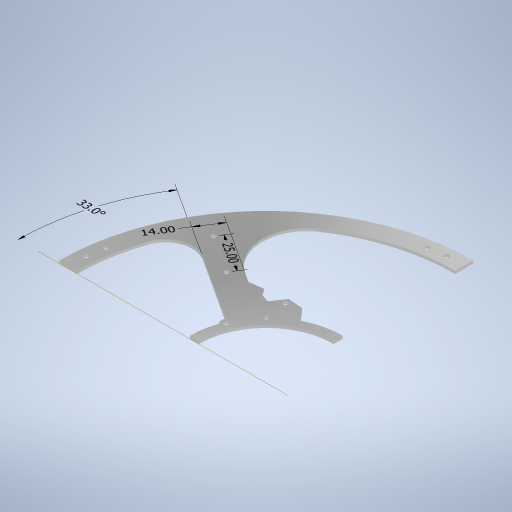
# Autodesk Inventor part: body_plate
Saved by Autodesk Inventor 2024.1 (Build 281209000, 209)
## iProperties
Created: 2024-08-02
Part Number: body_plate
Material: アルミニウム 6061
Document SubType Name: Sheet Metal
Designer: hibik
Density: 2.7 g/cm^3
Appearance: アルミニウム - フラット
Sheet Metal Rule: Default_mm
Author: hibik
Autodesk Inventor part; units mm, degrees
ref_plane "YZ Plane" through (0, 0, 0) normal (1, 0, 0) x (0, 1, 0)
ref_plane "XZ Plane" through (0, 0, 0) normal (0, 1, 0) x (-1, 0, 0)
ref_plane "XY Plane" through (0, 0, 0) normal (0, 0, 1) x (1, 0, 0)
sketch "スケッチ1" plane through (0, 0, 0) normal (0, 1, 0) x (-1, 0, 0)
  circle A0 centre (0, 0) radius 67
  circle A1 centre (0, 0) radius 62
  circle A2 centre (0, 0) radius 115
  circle A3 centre (0, 0) radius 105
  dimension "d0" = 134
  dimension "d1" = 124
  dimension "d2" = 230
  dimension "d5" = 210
  constraints: 4 centre point, 4 coincident
  measures "d0" diameter of A0
  measures "d1" diameter of A1
  measures "d2" diameter of A2
  measures "d5" diameter of A3
extrude "押し出し1" add sketch "スケッチ1" along normal blind 1.5
sketch "スケッチ2" plane through (0, 0, 0) normal (0, -1, 0) x (1, 0, 0)
  line L0 (40.8211, -35.6706) -> (45.1461, -32.6728) projected
  line L1 (45.1461, -32.6728) -> (44.7842, -28.2962) projected
  arc A0 (44.7842, -28.2962) -> (43.4491, -27.9248) centre (43.6139, -29.918) ccw projected
  line L2 (43.4491, -27.9248) -> (41.9542, -28.0485) projected
  arc A1 (41.9542, -28.0485) -> (38.889, -32.5383) centre (42.2426, -31.5365) ccw projected
  line L3 (38.889, -32.5383) -> (39.4183, -34.3101) projected
  arc A2 (39.4183, -34.3101) -> (40.8211, -35.6706) centre (41.3346, -33.7377) ccw projected
  circle A3 centre (42.2426, -31.5365) radius 1.35 projected
  arc A4 (20.2759, -44.9821) -> (16.4994, -41.7824) centre (16.7878, -45.2705) ccw projected
  line L4 (20.2759, -44.9821) -> (19.699, -38.0059) projected
  arc A5 (19.699, -38.0059) -> (15.9225, -34.8062) centre (16.2109, -38.2943) ccw projected
  line L5 (15.9225, -34.8062) -> (12.4344, -35.0947) projected
  line L6 (12.4344, -35.0947) -> (13.0113, -42.0709) projected
  line L7 (13.0113, -42.0709) -> (16.4994, -41.7824) projected
  circle A6 centre (16.2109, -38.2943) radius 1.35 projected
  line L8 (-32.6728, -45.1461) -> (-28.2962, -44.7842) projected
  arc A7 (-28.2962, -44.7842) -> (-27.9248, -43.4491) centre (-29.918, -43.6139) ccw projected
  line L9 (-27.9248, -43.4491) -> (-28.0485, -41.9542) projected
  arc A8 (-28.0485, -41.9542) -> (-32.5383, -38.889) centre (-31.5365, -42.2426) ccw projected
  line L10 (-32.5383, -38.889) -> (-34.3101, -39.4183) projected
  arc A9 (-34.3101, -39.4183) -> (-35.6706, -40.8211) centre (-33.7377, -41.3346) ccw projected
  line L11 (-35.6706, -40.8211) -> (-32.6728, -45.1461) projected
  circle A10 centre (-31.5365, -42.2426) radius 1.35 projected
  arc A11 (-44.9821, -20.2759) -> (-41.7824, -16.4994) centre (-45.2705, -16.7878) ccw projected
  line L12 (-44.9821, -20.2759) -> (-38.0059, -19.699) projected
  arc A12 (-38.0059, -19.699) -> (-34.8062, -15.9225) centre (-38.2943, -16.2109) ccw projected
  line L13 (-34.8062, -15.9225) -> (-35.0947, -12.4344) projected
  line L14 (-35.0947, -12.4344) -> (-42.0709, -13.0113) projected
  line L15 (-42.0709, -13.0113) -> (-41.7824, -16.4994) projected
  circle A13 centre (-38.2943, -16.2109) radius 1.35 projected
  arc A14 (-20.2759, 44.9821) -> (-16.4994, 41.7824) centre (-16.7878, 45.2705) ccw projected
  line L16 (-20.2759, 44.9821) -> (-19.699, 38.0059) projected
  arc A15 (-19.699, 38.0059) -> (-15.9225, 34.8062) centre (-16.2109, 38.2943) ccw projected
  line L17 (-15.9225, 34.8062) -> (-12.4344, 35.0947) projected
  line L18 (-12.4344, 35.0947) -> (-13.0113, 42.0709) projected
  line L19 (-13.0113, 42.0709) -> (-16.4994, 41.7824) projected
  circle A16 centre (-16.2109, 38.2943) radius 1.35 projected
  line L20 (35.6706, 40.8211) -> (32.6728, 45.1461) projected
  line L21 (32.6728, 45.1461) -> (28.2962, 44.7842) projected
  arc A17 (28.2962, 44.7842) -> (27.9248, 43.4491) centre (29.918, 43.6139) ccw projected
  line L22 (27.9248, 43.4491) -> (28.0485, 41.9542) projected
  arc A18 (28.0485, 41.9542) -> (32.5383, 38.889) centre (31.5365, 42.2426) ccw projected
  line L23 (32.5383, 38.889) -> (34.3101, 39.4183) projected
  arc A19 (34.3101, 39.4183) -> (35.6706, 40.8211) centre (33.7377, 41.3346) ccw projected
  circle A20 centre (31.5365, 42.2426) radius 1.35 projected
  circle A21 centre (-42.2426, 31.5365) radius 1.35 projected
  line L24 (-40.8211, 35.6706) -> (-45.1461, 32.6728) projected
  line L25 (-45.1461, 32.6728) -> (-44.7842, 28.2962) projected
  arc A22 (-44.7842, 28.2962) -> (-43.4491, 27.9248) centre (-43.6139, 29.918) ccw projected
  line L26 (-43.4491, 27.9248) -> (-41.9542, 28.0485) projected
  arc A23 (-41.9542, 28.0485) -> (-38.889, 32.5383) centre (-42.2426, 31.5365) ccw projected
  line L27 (-38.889, 32.5383) -> (-39.4183, 34.3101) projected
  arc A24 (-39.4183, 34.3101) -> (-40.8211, 35.6706) centre (-41.3346, 33.7377) ccw projected
  arc A25 (44.9821, 20.2759) -> (41.7824, 16.4994) centre (45.2705, 16.7878) ccw projected
  line L28 (44.9821, 20.2759) -> (38.0059, 19.699) projected
  arc A26 (38.0059, 19.699) -> (34.8062, 15.9225) centre (38.2943, 16.2109) ccw projected
  line L29 (34.8062, 15.9225) -> (35.0947, 12.4344) projected
  line L30 (35.0947, 12.4344) -> (42.0709, 13.0113) projected
  line L31 (42.0709, 13.0113) -> (41.7824, 16.4994) projected
  circle A27 centre (38.2943, 16.2109) radius 1.35 projected
  circle A28 centre (0, 0) radius 37.5
  line L32 (16.9004, -64.8335) -> (16.4816, -59.7692) projected
  arc A29 (16.9004, -64.8335) -> (45.2274, -49.4315) centre (0, 0) ccw projected
  line L33 (44.838, -44.7223) -> (45.2274, -49.4315) projected
  arc A30 (39.1412, -40.3701) -> (44.838, -44.7223) centre (44.986, -38.6241) ccw projected
  line L34 (36.9727, -33.1108) -> (39.1412, -40.3701) projected
  arc A31 (41.7893, -26.0553) -> (36.9727, -33.1108) centre (42.2426, -31.5365) ccw projected
  line L35 (45.2774, -25.7668) -> (41.7893, -26.0553) projected
  line L36 (45.2319, -25.2161) -> (45.2774, -25.7668) projected
  line L37 (45.2319, -25.2161) -> (29.6057, -11.9768) projected
  arc A32 (16.6771, -27.2363) -> (29.6057, -11.9768) centre (0, 0) ccw projected
  line L38 (16.6771, -27.2363) -> (40.2207, -47.1836) projected
  arc A33 (16.4816, -59.7692) -> (40.2207, -47.1836) centre (0, 0) ccw projected
  line L39 (-64.8335, -16.9004) -> (-59.7692, -16.4816) projected
  arc A34 (-64.8335, -16.9004) -> (-49.4315, -45.2274) centre (0, 0) ccw projected
  line L40 (-44.7223, -44.838) -> (-49.4315, -45.2274) projected
  arc A35 (-40.3701, -39.1412) -> (-44.7223, -44.838) centre (-38.6241, -44.986) ccw projected
  line L41 (-33.1108, -36.9727) -> (-40.3701, -39.1412) projected
  arc A36 (-26.0553, -41.7893) -> (-33.1108, -36.9727) centre (-31.5365, -42.2426) ccw projected
  line L42 (-25.9316, -43.2842) -> (-26.0553, -41.7893) projected
  line L43 (-23.3877, -43.0739) -> (-25.9316, -43.2842) projected
  line L44 (-23.3877, -43.0739) -> (-11.9768, -29.6057) projected
  arc A37 (-27.2363, -16.6771) -> (-11.9768, -29.6057) centre (0, 0) ccw projected
  line L45 (-27.2363, -16.6771) -> (-47.1836, -40.2207) projected
  arc A38 (-59.7692, -16.4816) -> (-47.1836, -40.2207) centre (0, 0) ccw projected
  line L46 (-16.9004, 64.8335) -> (-16.4816, 59.7692) projected
  arc A39 (-16.9004, 64.8335) -> (-45.2274, 49.4315) centre (0, 0) ccw projected
  line L47 (-44.838, 44.7223) -> (-45.2274, 49.4315) projected
  arc A40 (-39.1412, 40.3701) -> (-44.838, 44.7223) centre (-44.986, 38.6241) ccw projected
  line L48 (-36.9727, 33.1108) -> (-39.1412, 40.3701) projected
  arc A41 (-41.7893, 26.0553) -> (-36.9727, 33.1108) centre (-42.2426, 31.5365) ccw projected
  line L49 (-43.2842, 25.9316) -> (-41.7893, 26.0553) projected
  line L50 (-43.0739, 23.3877) -> (-43.2842, 25.9316) projected
  line L51 (-43.0739, 23.3877) -> (-29.6057, 11.9768) projected
  arc A42 (-16.6771, 27.2363) -> (-29.6057, 11.9768) centre (0, 0) ccw projected
  line L52 (-16.6771, 27.2363) -> (-40.2207, 47.1836) projected
  arc A43 (-16.4816, 59.7692) -> (-40.2207, 47.1836) centre (0, 0) ccw projected
  line L53 (64.8335, 16.9004) -> (59.7692, 16.4816) projected
  arc A44 (64.8335, 16.9004) -> (49.4315, 45.2274) centre (0, 0) ccw projected
  line L54 (44.7223, 44.838) -> (49.4315, 45.2274) projected
  arc A45 (40.3701, 39.1412) -> (44.7223, 44.838) centre (38.6241, 44.986) ccw projected
  line L55 (33.1108, 36.9727) -> (40.3701, 39.1412) projected
  arc A46 (26.0553, 41.7893) -> (33.1108, 36.9727) centre (31.5365, 42.2426) ccw projected
  line L56 (25.9316, 43.2842) -> (26.0553, 41.7893) projected
  line L57 (23.3877, 43.0739) -> (25.9316, 43.2842) projected
  line L58 (23.3877, 43.0739) -> (11.9768, 29.6057) projected
  arc A47 (27.2363, 16.6771) -> (11.9768, 29.6057) centre (0, 0) ccw projected
  line L59 (27.2363, 16.6771) -> (47.1836, 40.2207) projected
  arc A48 (59.7692, 16.4816) -> (47.1836, 40.2207) centre (0, 0) ccw projected
  circle A49 centre (0, 0) radius 42.5
  line L60 (10.8533, -40.2425) -> (13.0113, -42.0709) projected
  line L61 (6.3617, -40.6139) -> (6.5265, -42.6071) projected
  line L62 (-40.6139, -6.3617) -> (-42.6071, -6.5265) projected
  line L63 (-6.3617, 40.6139) -> (-6.5265, 42.6071) projected
  line L64 (31.4411, 5.6032) -> (42.6071, 6.5265) projected
  line L65 (40.8211, -35.6706) -> (38.2663, -37.4414)
  line L66 (44.7842, -28.2962) -> (44.4766, -24.5762)
  line L67 (35.6706, 40.8211) -> (37.4414, 38.2663)
  line L68 (28.2962, 44.7842) -> (24.5762, 44.4766)
  line L69 (-40.8211, 35.6706) -> (-38.2663, 37.4414)
  line L70 (-44.7842, 28.2962) -> (-44.4766, 24.5762)
  line L71 (-35.6706, -40.8211) -> (-37.4414, -38.2663)
  line L72 (-28.2962, -44.7842) -> (-24.5762, -44.4766)
  line L73 (-25.2161, -45.2319) -> (-23.3877, -43.0739) projected
  line L74 (-45.2319, 25.2161) -> (-43.0739, 23.3877) projected
  line L75 (25.2161, 45.2319) -> (23.3877, 43.0739) projected
  circle A50 centre (-16.2109, 38.2943) radius 3
  circle A51 centre (-38.2943, -16.2109) radius 3
  circle A52 centre (16.2109, -38.2943) radius 3
  circle A53 centre (38.2943, 16.2109) radius 3
  point P0 (40.1725, 13.8716)
  point P1 (37.922, 19.1878)
  point P2 (-13.8716, 40.1725)
  point P3 (-19.1878, 37.922)
  point P4 (-25.0517, 34.3317)
  point P5 (-37.9803, 19.0722)
  point P6 (-40.1725, -13.8716)
  point P7 (-37.922, -19.1878)
  point P8 (-34.3317, -25.0517)
  point P9 (-19.0722, -37.9803)
  point P10 (13.8716, -40.1725)
  point P11 (19.1878, -37.922)
  point P12 (25.0517, -34.3317)
  point P13 (37.9803, -19.0722)
  point P14 (19.0722, 37.9803)
  point P15 (34.3317, 25.0517)
  dimension "d6" = 75
  dimension "d7" = 85
  dimension "d10" = 360
  dimension "d12" = 6
  dimension "d13" = 6
  dimension "d14" = 6
  dimension "d15" = 6
  constraints: 16 end point, 6 centre point, 6 coincident, 2 collinear, 2 point on line, 25 other
  measures "d6" diameter of A28
  measures "d7" diameter of A49
  measures "d12" diameter of A50
  measures "d13" diameter of A51
  measures "d14" diameter of A52
  measures "d15" diameter of A53
extrude "押し出し2" add sketch "スケッチ2" against normal up to surface (1.5 mm away) contours A2 L3 A1 L2 A0 L1 L0 | L65 L34 A31 L35 L66 A0 L2 A1 L3 A2 | L34 A30 L33 A29 L32 A33 L38 A49 L37 L66 L35 A31 | A49 L38 A28 L37 | L37 A28 L64 A49 | A49 A5 L5 A28 L38 | A49 A52 L6 A28 L5 A5 | L64 A28 L30 A49 | A52 A49 A6 | A49 A6 A52 | L30 A28 L29 A26 A49 A53 | L6 A49 L44 A28 | A53 A49 A27 | A49 A27 A53 | L44 A49 L45 A28 | A28 L59 A49 A26 L29 | L45 A49 A12 L13 A28 | L44 L43 L42 A36 L41 A35 L40 A34 L39 A38 L45 A49 | A28 L58 A49 L59 | L13 A12 A49 A51 L14 A28 | L73 L72 A7 L9 A8 L10 A9 L71 L41 A36 L42 L43 | A28 L18 A49 L58 | A49 L58 L57 L56 A46 L55 A45 L54 A44 L53 A48 L59 | L14 A49 L51 A28 | A28 L17 A15 A49 A50 L18 | L51 A49 L52 A28 | A51 A49 A13 | A49 A13 A51 | L8 L11 A9 L10 A8 L9 A7 | A28 L52 A49 A15 L17 | L75 L68 A17 L22 A18 L23 A19 L67 L55 A46 L56 L57 | L51 L50 L49 A41 L48 A40 L47 A39 L46 A43 L52 A49 | A50 A49 A16 | A49 A16 A50 | L74 L70 A22 L26 A23 L27 A24 L69 L48 A41 L49 L50 | L21 L20 A19 L23 A18 L22 A17 | L25 L24 A24 L27 A23 L26 A22
sketch "スケッチ3" plane through (0, 0, 0) normal (0, -1, 0) x (1, 0, 0)
  line L0 (-63.0578, 84.2479) -> (51.3164, -91.8729)
  line L1 (51.3164, -91.8729) -> (63.0578, -84.2479) construction
  line L2 (63.0578, -84.2479) -> (-51.3164, 91.8729)
  line L3 (-51.3164, 91.8729) -> (-63.0578, 84.2479) construction
  line L4 (-63.0578, 84.2479) -> (63.0578, -84.2479) construction
  line L5 (51.3164, -91.8729) -> (-51.3164, 91.8729) construction
  line L6 (91.8729, 51.3164) -> (-84.2479, -63.0578)
  line L7 (-84.2479, -63.0578) -> (-91.8729, -51.3164) construction
  line L8 (-91.8729, -51.3164) -> (84.2479, 63.0578)
  line L9 (84.2479, 63.0578) -> (91.8729, 51.3164) construction
  circle A0 centre (0, 0) radius 105 projected
  line L10 (91.8729, 51.3164) -> (-91.8729, -51.3164) construction
  line L11 (-84.2479, -63.0578) -> (84.2479, 63.0578) construction
  line L12 (0, -161) -> (0, 161) projected
  circle A1 centre (0, 0) radius 67 projected
  arc A2 (-44.4604, -43.2119) -> (40.2207, -47.1836) centre (0, 0) ccw projected
  arc A3 (-40.3701, -39.1412) -> (-44.4604, -43.2119) centre (-38.6241, -44.986) ccw projected
  line L13 (-40.3701, -39.1412) -> (-37.4414, -38.2663) projected
  line L14 (-37.4414, -38.2663) -> (-32.6728, -45.1461) projected
  line L15 (-32.6728, -45.1461) -> (-24.5762, -44.4766) projected
  line L16 (-24.5762, -44.4766) -> (-19.0722, -37.9803) projected
  arc A4 (-19.0722, -37.9803) -> (13.8716, -40.1725) centre (0, 0) ccw projected
  arc A5 (13.8716, -40.1725) -> (19.1878, -37.922) centre (16.2109, -38.2943) ccw projected
  arc A6 (19.1878, -37.922) -> (25.0517, -34.3317) centre (0, 0) ccw projected
  line L17 (25.0517, -34.3317) -> (40.2207, -47.1836) projected
  arc A7 (39.1412, -40.3701) -> (43.2119, -44.4604) centre (44.986, -38.6241) ccw projected
  line L18 (39.1412, -40.3701) -> (38.2663, -37.4414) projected
  line L19 (38.2663, -37.4414) -> (45.1461, -32.6728) projected
  line L20 (45.1461, -32.6728) -> (44.4766, -24.5762) projected
  line L21 (44.4766, -24.5762) -> (37.9803, -19.0722) projected
  arc A8 (37.9803, -19.0722) -> (40.1725, 13.8716) centre (0, 0) ccw projected
  arc A9 (40.1725, 13.8716) -> (37.922, 19.1878) centre (38.2943, 16.2109) ccw projected
  arc A10 (37.922, 19.1878) -> (34.3317, 25.0517) centre (0, 0) ccw projected
  arc A11 (-13.8716, 40.1725) -> (-19.1878, 37.922) centre (-16.2109, 38.2943) ccw projected
  arc A12 (-19.1878, 37.922) -> (-25.0517, 34.3317) centre (0, 0) ccw projected
  line L22 (-25.0517, 34.3317) -> (-40.2207, 47.1836) projected
  arc A13 (44.4604, 43.2119) -> (-40.2207, 47.1836) centre (0, 0) ccw projected
  circle A14 centre (0, 0) radius 37.5 projected
  circle A15 centre (42.2426, -31.5365) radius 1.35 projected
  circle A16 centre (16.2109, -38.2943) radius 1.35 projected
  circle A17 centre (-38.2943, -16.2109) radius 1.35 projected
  circle A18 centre (-16.2109, 38.2943) radius 1.35 projected
  circle A19 centre (38.2943, 16.2109) radius 1.35 projected
  circle A20 centre (-42.2426, 31.5365) radius 1.35 projected
  circle A21 centre (-31.5365, -42.2426) radius 1.35 projected
  arc A22 (-39.1412, 40.3701) -> (-43.2119, 44.4604) centre (-44.986, 38.6241) ccw projected
  line L23 (-39.1412, 40.3701) -> (-38.2663, 37.4414) projected
  line L24 (-38.2663, 37.4414) -> (-45.1461, 32.6728) projected
  line L25 (-45.1461, 32.6728) -> (-44.4766, 24.5762) projected
  line L26 (-44.4766, 24.5762) -> (-37.9803, 19.0722) projected
  arc A23 (-37.9803, 19.0722) -> (-40.1725, -13.8716) centre (0, 0) ccw projected
  arc A24 (-40.1725, -13.8716) -> (-37.922, -19.1878) centre (-38.2943, -16.2109) ccw projected
  arc A25 (-37.922, -19.1878) -> (-34.3317, -25.0517) centre (0, 0) ccw projected
  line L27 (-34.3317, -25.0517) -> (-47.1836, -40.2207) projected
  arc A26 (-43.2119, 44.4604) -> (-47.1836, -40.2207) centre (0, 0) ccw projected
  circle A27 centre (0, 0) radius 67 projected
  line L28 (34.3317, 25.0517) -> (47.1836, 40.2207) projected
  arc A28 (43.2119, -44.4604) -> (47.1836, 40.2207) centre (0, 0) ccw projected
  arc A29 (40.3701, 39.1412) -> (44.4604, 43.2119) centre (38.6241, 44.986) ccw projected
  line L29 (40.3701, 39.1412) -> (37.4414, 38.2663) projected
  line L30 (37.4414, 38.2663) -> (32.6728, 45.1461) projected
  line L31 (32.6728, 45.1461) -> (24.5762, 44.4766) projected
  line L32 (24.5762, 44.4766) -> (19.0722, 37.9803) projected
  arc A30 (19.0722, 37.9803) -> (-13.8716, 40.1725) centre (0, 0) ccw projected
  point P0 (42.1618, -52.0709)
  point P1 (30.4204, -59.6959)
  point P2 (51.1892, -91.677)
  point P3 (62.9306, -84.052)
  point P4 (18.0575, -40.6587)
  point P5 (27.681, -55.4776)
  point P6 (-52.0709, -42.1618)
  point P7 (-59.6959, -30.4204)
  point P8 (-91.677, -51.1892)
  point P9 (-84.052, -62.9306)
  point P10 (-40.6587, -18.0575)
  point P11 (-55.4776, -27.681)
  point P12 (-42.1618, 52.0709)
  point P13 (-30.4204, 59.6959)
  point P14 (-51.1892, 91.677)
  point P15 (-62.9306, 84.052)
  point P16 (-18.0575, 40.6587)
  point P17 (-27.681, 55.4776)
  point P18 (40.6587, 18.0575)
  point P19 (55.4776, 27.681)
  point P20 (52.0709, 42.1618)
  point P21 (59.6959, 30.4204)
  point P22 (91.677, 51.1892)
  point P23 (84.052, 62.9306)
  dimension "d18" = 14
  dimension "d19" = 33
  constraints: 24 end point, 4 midpoint, 4 parallel, 4 perpendicular, 2 tangent
  measures "d18" distance between parallel lines of L2 L0
  measures "d19" angle of L0 L12
extrude "押し出し3" add sketch "スケッチ3" against normal up to surface (1.5 mm away) contours A0 L2 A1 L0 | L8 A1 L6 A0 | A13 L2 A11 A12 L22 L0 | L0 L22 A13 | L8 A24 A25 L27 L6 A26 | A0 L6 A1 L8 | L6 L27 A26 | L0 A1 L2 A0 | A28 L6 A9 A10 L28 L8 | L8 L28 A28 | L0 A5 A6 L17 L2 A2 | L2 L17 A2
sketch "スケッチ4" plane through (0, 0, 0) normal (0, -1, 0) x (1, 0, 0)
  arc A0 (52.0709, 42.1618) -> (-30.4204, 59.6959) centre (0, 0) ccw projected
  line L0 (-30.4204, 59.6959) -> (-51.1892, 91.677) projected
  arc A1 (84.052, 62.9306) -> (-51.1892, 91.677) centre (0, 0) ccw projected
  line L1 (84.052, 62.9306) -> (52.0709, 42.1618) projected
  line L2 (59.6959, 30.4204) -> (91.677, 51.1892) projected
  arc A2 (62.9306, -84.052) -> (91.677, 51.1892) centre (0, 0) ccw projected
  line L3 (62.9306, -84.052) -> (42.1618, -52.0709) projected
  arc A3 (42.1618, -52.0709) -> (59.6959, 30.4204) centre (0, 0) ccw projected
  arc A4 (-42.1618, 52.0709) -> (-59.6959, -30.4204) centre (0, 0) ccw projected
  line L4 (-59.6959, -30.4204) -> (-91.677, -51.1892) projected
  arc A5 (-62.9306, 84.052) -> (-91.677, -51.1892) centre (0, 0) ccw projected
  line L5 (-62.9306, 84.052) -> (-42.1618, 52.0709) projected
  circle A6 centre (0, 0) radius 115 projected
  arc A7 (-43.2119, 44.4604) -> (-55.4776, -27.681) centre (0, 0) ccw projected
  arc A8 (-39.1412, 40.3701) -> (-43.2119, 44.4604) centre (-44.986, 38.6241) ccw projected
  line L6 (-39.1412, 40.3701) -> (-38.2663, 37.4414) projected
  line L7 (-38.2663, 37.4414) -> (-45.1461, 32.6728) projected
  line L8 (-45.1461, 32.6728) -> (-44.4766, 24.5762) projected
  line L9 (-44.4766, 24.5762) -> (-37.9803, 19.0722) projected
  arc A9 (-37.9803, 19.0722) -> (-40.1725, -13.8716) centre (0, 0) ccw projected
  arc A10 (-40.1725, -13.8716) -> (-40.6587, -18.0575) centre (-38.2943, -16.2109) ccw projected
  line L10 (-40.6587, -18.0575) -> (-55.4776, -27.681) projected
  arc A11 (-40.3701, -39.1412) -> (-44.4604, -43.2119) centre (-38.6241, -44.986) ccw projected
  line L11 (-40.3701, -39.1412) -> (-37.4414, -38.2663) projected
  line L12 (-37.4414, -38.2663) -> (-32.6728, -45.1461) projected
  line L13 (-32.6728, -45.1461) -> (-24.5762, -44.4766) projected
  line L14 (-24.5762, -44.4766) -> (-19.0722, -37.9803) projected
  arc A12 (-19.0722, -37.9803) -> (13.8716, -40.1725) centre (0, 0) ccw projected
  arc A13 (13.8716, -40.1725) -> (18.0575, -40.6587) centre (16.2109, -38.2943) ccw projected
  line L15 (18.0575, -40.6587) -> (27.681, -55.4776) projected
  arc A14 (-44.4604, -43.2119) -> (27.681, -55.4776) centre (0, 0) ccw projected
  arc A15 (39.1412, -40.3701) -> (43.2119, -44.4604) centre (44.986, -38.6241) ccw projected
  line L16 (39.1412, -40.3701) -> (38.2663, -37.4414) projected
  line L17 (38.2663, -37.4414) -> (45.1461, -32.6728) projected
  line L18 (45.1461, -32.6728) -> (44.4766, -24.5762) projected
  line L19 (44.4766, -24.5762) -> (37.9803, -19.0722) projected
  arc A16 (37.9803, -19.0722) -> (40.1725, 13.8716) centre (0, 0) ccw projected
  arc A17 (40.1725, 13.8716) -> (40.6587, 18.0575) centre (38.2943, 16.2109) ccw projected
  line L20 (40.6587, 18.0575) -> (55.4776, 27.681) projected
  arc A18 (43.2119, -44.4604) -> (55.4776, 27.681) centre (0, 0) ccw projected
  circle A19 centre (0, 0) radius 37.5 projected
  circle A20 centre (42.2426, -31.5365) radius 1.35 projected
  circle A21 centre (16.2109, -38.2943) radius 1.35 projected
  circle A22 centre (-38.2943, -16.2109) radius 1.35 projected
  circle A23 centre (-16.2109, 38.2943) radius 1.35 projected
  circle A24 centre (38.2943, 16.2109) radius 1.35 projected
  circle A25 centre (-42.2426, 31.5365) radius 1.35 projected
  circle A26 centre (-31.5365, -42.2426) radius 1.35 projected
  circle A27 centre (31.5365, 42.2426) radius 1.35 projected
  arc A28 (40.3701, 39.1412) -> (44.4604, 43.2119) centre (38.6241, 44.986) ccw projected
  line L21 (40.3701, 39.1412) -> (37.4414, 38.2663) projected
  line L22 (37.4414, 38.2663) -> (32.6728, 45.1461) projected
  line L23 (32.6728, 45.1461) -> (24.5762, 44.4766) projected
  line L24 (24.5762, 44.4766) -> (19.0722, 37.9803) projected
  arc A29 (19.0722, 37.9803) -> (-13.8716, 40.1725) centre (0, 0) ccw projected
  arc A30 (-13.8716, 40.1725) -> (-18.0575, 40.6587) centre (-16.2109, 38.2943) ccw projected
  line L25 (-18.0575, 40.6587) -> (-27.681, 55.4776) projected
  arc A31 (44.4604, 43.2119) -> (-27.681, 55.4776) centre (0, 0) ccw projected
  line L26 (30.4204, -59.6959) -> (51.1892, -91.677) projected
  arc A32 (-84.052, -62.9306) -> (51.1892, -91.677) centre (0, 0) ccw projected
  line L27 (-84.052, -62.9306) -> (-52.0709, -42.1618) projected
  arc A33 (-52.0709, -42.1618) -> (30.4204, -59.6959) centre (0, 0) ccw projected
  line L28 (30.4204, -59.6959) -> (27.681, -55.4776)
  line L29 (-52.0709, -42.1618) -> (-44.4604, -43.2119)
  line L30 (42.1618, -52.0709) -> (43.2119, -44.4604)
  line L31 (59.6959, 30.4204) -> (55.4776, 27.681)
  line L32 (52.0709, 42.1618) -> (44.4604, 43.2119)
  line L33 (-30.4204, 59.6959) -> (-27.681, 55.4776)
  line L34 (-42.1618, 52.0709) -> (-43.2119, 44.4604)
  line L35 (-59.6959, -30.4204) -> (-55.4776, -27.681)
  circle A34 centre (62.9003, 40.8479) radius 1.3
  line L36 (62.9003, 40.8479) -> (0, 0) construction
  line L37 (62.9003, 40.8479) -> (64.3271, 38.6509) construction
  circle A35 centre (83.8671, 54.4639) radius 1.3
  line L38 (62.9003, 40.8479) -> (83.8671, 54.4639) construction
  circle A36 centre (-54.4639, 83.8671) radius 1.3
  circle A37 centre (-40.8479, 62.9003) radius 1.3
  circle A38 centre (-83.8671, -54.4639) radius 1.3
  circle A39 centre (-62.9003, -40.8479) radius 1.3
  circle A40 centre (54.4639, -83.8671) radius 1.3
  circle A41 centre (40.8479, -62.9003) radius 1.3
  point P0 (-30.4204, 59.6959)
  point P1 (44.4604, 43.2119)
  point P2 (-59.6959, -30.4204)
  dimension "d24" = 360
  dimension "d34" = 2.6
  dimension "d35" = 7
  dimension "d36" = 7
  dimension "d37" = 75
  dimension "d39" = 25
  dimension "d42" = 360
  constraints: 22 end point, 8 centre point, 2 coincident, 2 collinear, 1 equal radius, 1 perpendicular, 44 other
  measures "d34" diameter of A34
  measures "d35" distance from line of L1 L36.start
  measures "d36" distance from line of L2 L36.start
  measures "d37" distance from line of point (0, 0) L37
  measures "d39" distance from line of L38.end L37
extrude "押し出し4" cut sketch "スケッチ4" against normal through all contours L32 A31 L33 A0 | A3 L30 A18 L31 | L34 A7 L35 A4 | A14 L28 A33 L29 | A34 | A35 | A36 | A37 | A38 | A39 | A40 | A41
fillet "フィレット1" radius 25 4 edges at (62.9306, 0.75, -84.052) (84.052, 0.75, 62.9306) (-62.9306, 0.75, 84.052) (-84.052, 0.75, -62.9306)
fillet "フィレット2" radius 15 4 edges at (91.677, 0.75, 51.1892) (51.1892, 0.75, -91.677) (-91.677, 0.75, -51.1892) (-51.1892, 0.75, 91.677)
sketch "スケッチ5" plane through (0, 0, 0) normal (0, -1, 0) x (1, 0, 0)
  line L0 (30, 30) -> (-30, 30) construction
  line L1 (-30, 30) -> (-30, -30) construction
  line L2 (-30, -30) -> (30, -30) construction
  line L3 (30, -30) -> (30, 30) construction
  line L4 (30, 30) -> (-30, -30) construction
  line L5 (-30, 30) -> (30, -30) construction
  circle A0 centre (-30, 30) radius 1.3
  circle A1 centre (30, 30) radius 1.3
  circle A2 centre (30, -30) radius 1.3
  circle A3 centre (-30, -30) radius 1.3
  point P0 (0, 0)
  dimension "d30" = 2.6
  dimension "d31" = 60
  constraints: 12 end point, 4 centre point, 4 coincident, 3 equal radius, 2 midpoint, 2 parallel, 2 perpendicular, 1 horizontal
  measures "d30" diameter of A0
  measures "d31" distance of L0.start L0.end
extrude "押し出し5" cut sketch "スケッチ5" against normal through all
sketch "スケッチ6" plane through (0, 1.5, 0) normal (0, 1, 0) x (1, 0, 0)
  line L0 (0, 139.1279) -> (158.6637, 139.1279)
  line L1 (158.6637, 139.1279) -> (158.6637, -140)
  line L2 (158.6637, -140) -> (0, -140)
  line L3 (0, -140) -> (0, 139.1279)
  line L4 (-207.7572, 0) -> (158.6637, 0)
  line L5 (158.6637, 0) -> (158.6637, -140)
  line L6 (158.6637, -140) -> (-207.7572, -140)
  line L7 (-207.7572, -140) -> (-207.7572, 0)
  line L8 (0, 194.9535) -> (0, -195.8256) projected
  line L9 (-281.0413, 0) -> (231.9478, 0) projected
  point P0 (0, 0)
  point P1 (0, 0)
  constraints: 16 end point, 4 parallel, 3 collinear, 2 horizontal, 2 perpendicular, 1 point on line
extrude "押し出し6" cut sketch "スケッチ6" against normal through all
sketch "スケッチ7" plane through (0, 1.5, 0) normal (0, 1, 0) x (1, 0, 0)
  line L0 (0, 0) -> (-109.5814, 9.5871) construction
  line L1 (0, 0) -> (-108.3289, 19.1013) construction
  line L2 (0, 0) -> (-19.1013, 108.3289) construction
  line L3 (0, 0) -> (-9.5871, 109.5814) construction
  line L4 (0, 161) -> (0, -161) projected
  line L5 (-161, 0) -> (161, 0) projected
  circle A0 centre (0, 0) radius 110 construction
  circle A1 centre (-9.5871, 109.5814) radius 1.5
  circle A2 centre (-19.1013, 108.3289) radius 1.5
  circle A3 centre (-108.3289, 19.1013) radius 1.5
  circle A4 centre (-109.5814, 9.5871) radius 1.5
  dimension "d46" = 5
  dimension "d47" = 5
  dimension "d48" = 5
  dimension "d49" = 5
  dimension "d50" = 220
  dimension "d51" = 3
  constraints: 8 end point, 5 centre point, 5 coincident, 4 point on circle, 3 equal radius
  measures "d46" angle of L3 L4
  measures "d47" angle of L2 L3
  measures "d48" angle of L5 L0
  measures "d49" angle of L1 L0
  measures "d50" diameter of A0
  measures "d51" diameter of A1
extrude "押し出し7" cut sketch "スケッチ7" against normal through all
equation "\"d35\" = d36"
equation "\"BendRadius\" = Thickness"
equation "\"BendReliefWidth\" = Thickness"
equation "\"BendReliefDepth\" = 0.5 * Thickness"
equation "\"CornerReliefSize\" = 4 * Thickness"
equation "\"MinimumRemnant\" = 2 * Thickness"
equation "\"TransitionRadius\" = BendRadius"
equation "\"JacobiRadiusSize\" = BendRadius"
equation "\"GapSize\" = Thickness"
equation "\"Thickness\" = 1.5"
